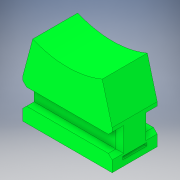
# Autodesk Inventor part: Wood Rail Selector
Saved by Autodesk Inventor 2018 (Build 220112000, 112)
## iProperties
Created: 2017-12-04
Part Number: Wood Rail Selector
Material: Generic
Document SubType Name: Modeling
Designer: Andrew
Density: 1 g/cm^3
Appearance: Default(1)
Author: Andrew
Autodesk Inventor part; units mm, degrees
ref_plane "YZ Plane" through (0, 0, 0) normal (1, 0, 0) x (0, 1, 0)
ref_plane "XZ Plane" through (0, 0, 0) normal (0, 1, 0) x (-1, 0, 0)
ref_plane "XY Plane" through (0, 0, 0) normal (0, 0, 1) x (1, 0, 0)
sketch "Sketch1" plane through (0, 0, 0) normal (1, 0, 0) x (0, 1, 0)
  line L0 (11.2875, 4.8006) -> (11.2875, -4.8006)
  line L1 (11.2875, -4.8006) -> (1.7625, -4.8006)
  line L2 (1.7625, -4.8006) -> (1.7625, -3.175)
  line L3 (1.7625, -3.175) -> (-1.7625, -3.175)
  line L4 (-1.7625, -3.175) -> (-1.7625, -4.8006)
  line L5 (-1.7625, -4.8006) -> (-4.9375, -4.8006)
  line L6 (-4.9375, -4.8006) -> (-4.9375, 4.8006)
  line L7 (-4.9375, 4.8006) -> (-1.7625, 4.8006)
  line L8 (-1.7625, 4.8006) -> (-1.7625, 3.175)
  line L9 (-1.7625, 3.175) -> (1.7625, 3.175)
  line L10 (1.7625, 3.175) -> (1.7625, 4.8006)
  line L11 (-8.1825, 0) -> (14.5325, 0) projected
  line L12 (11.2875, 4.8006) -> (1.7625, 4.8006)
  line L13 (-3.6774, 2.54) -> (-3.0226, 2.54)
  line L14 (-3.0226, 2.54) -> (-3.0226, -2.54)
  line L15 (-3.0226, -2.54) -> (-3.6774, -2.54)
  line L16 (-3.6774, -2.54) -> (-3.6774, 2.54)
  line L17 (-3.6774, 2.54) -> (-3.0226, -2.54) construction
  line L18 (-3.0226, 2.54) -> (-3.6774, -2.54) construction
  point P0 (0, 0)
  point P1 (0, -3.175)
  point P2 (-3.35, 0)
  point P3 (-3.35, 0)
  point P4 (-3.35, 4.8006)
  dimension "d0" = 3.525
  dimension "d1" = 9.525
  dimension "d2" = 6.35
  dimension "d3" = 1.6256
  dimension "d4" = 3.175
  dimension "d14" = 0.6548
  dimension "d15" = 5.08
  constraints: 36 end point, 8 perpendicular, 8 point on line, 5 midpoint, 2 horizontal, 2 parallel, 2 vertical alignment, 1 vertical, 2 other
  measures "d0" distance of L2.end L3.end
  measures "d1" distance of L0.end L1.end
  measures "d2" distance between parallel lines of L9 L3
  measures "d3" distance of L9.end L10.end
  measures "d4" distance of L4.end L5.end
  measures "d14" distance of L14.end L15.end
  measures "d15" distance of L13.end L14.end
extrude "Extrusion1" add sketch "Sketch1" along normal mid plane 19.05 contours L0 L11 L14 L13 L16 L6 L7 L8 L9 L10 L12 | L0 L1 L2 L3 L4 L5 L6 L11 L16 L15 L14
sketch "Sketch2" plane through (0, 0, 0) normal (0, 0, 1) x (1, 0, 0)
  line L0 (-9.525, 1.7625) -> (-9.525, 11.2875) construction
  line L1 (9.525, 11.2875) -> (9.525, 1.7625) construction
  line L2 (-9.525, 3.3881) -> (-7.4084, 11.2875)
  line L3 (9.525, 11.2875) -> (-9.525, 11.2875) projected
  line L4 (7.4084, 11.2875) -> (9.525, 3.3881)
  line L5 (9.525, 1.7625) -> (9.525, 11.2875) projected
  arc A0 (-7.4084, 11.2875) -> (7.4084, 11.2875) centre (0, 28.838) ccw
  line L6 (-7.4084, 11.2875) -> (-9.525, 11.2875)
  line L7 (-9.525, 11.2875) -> (-9.525, 3.3881)
  line L8 (-9.525, 11.2875) -> (-9.525, 1.7625) projected
  line L9 (9.525, 3.3881) -> (9.525, 11.2875)
  line L10 (9.525, 11.2875) -> (7.4084, 11.2875)
  line L11 (7.4084, 11.2875) -> (-7.4084, 11.2875)
  line L12 (0, 34.3956) -> (0, -5.7326) construction
  point P0 (0, 0)
  dimension "d7" = 19.05
  dimension "d8" = 1.6256
  dimension "d9" = 15
  constraints: 14 end point, 4 point on line, 3 collinear, 2 point on circle, 1 centre point, 1 parallel, 1 perpendicular, 1 other
  measures "d7" radius of A0
  measures "d8" distance of L4.end L1.end
  measures "d9" angle of L1 L4
extrude "Extrusion2" cut sketch "Sketch2" along normal up to next
extrude "Extrusion3" cut sketch "Sketch2" against normal up to next
derived "Conductive Rail.ipt"
derived "Wood Rail.ipt"
chamfer "Chamfer1" distance 0.8128 angle 45 12 edges at (-9.525, -1.7625, 3.9878) (9.525, -1.7625, 3.9878) (9.525, 1.7625, 3.9878) (-9.525, 1.7625, 3.9878) (9.525, -1.7625, -3.9878) (9.525, 1.7625, -3.9878) (-9.525, 1.7625, -3.9878) (-9.525, -1.7625, -3.9878) (-9.525, 0, 3.175) (-9.525, 0, -3.175) (9.525, 0, -3.175) (9.525, 0, 3.175)
equation "\"d14\" = springSteelThickness"
equation "\"d15\" = springSteelWidth"
equation "\"springSteelThickness\" = 0.6548"
equation "\"springSteelWidth\" = 5.08"
body "Solid1"
